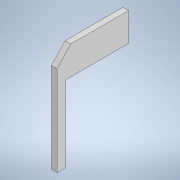
# Autodesk Inventor part: GripperServoAtt
Saved by Autodesk Inventor 2020 (Build 240168000, 168)
## iProperties
Created: 2020-01-21
Part Number: GripperServoAtt
Material: Generic
Document SubType Name: Modeling
Designer: tdmp4
Density: 1 g/cm^3
Appearance: Default
Author: tdmp4
Autodesk Inventor part; units mm, degrees
ref_plane "YZ Plane" through (0, 0, 0) normal (1, 0, 0) x (0, 1, 0)
ref_plane "XZ Plane" through (0, 0, 0) normal (0, 1, 0) x (-1, 0, 0)
ref_plane "XY Plane" through (0, 0, 0) normal (0, 0, 1) x (1, 0, 0)
sketch "Sketch1" plane through (0, 0, 0) normal (1, 0, 0) x (0, 1, 0)
  line L0 (0, 0) -> (25.4, 0)
  line L1 (25.4, 0) -> (25.4, -9.525)
  line L2 (25.4, -9.525) -> (0, -9.525)
  line L3 (0, -9.525) -> (0, 0)
  line L4 (25.4, -9.525) -> (35.5298, -9.525)
  line L5 (35.5298, -9.525) -> (35.5298, -29.845)
  line L6 (25.4, -9.525) -> (25.4, -24.4288)
  line L7 (25.4, -24.4288) -> (25.4, -29.845)
  line L8 (35.5298, -29.845) -> (26.0048, -29.845)
  line L9 (26.0048, -29.845) -> (26.0048, -80.645)
  line L10 (26.0048, -80.645) -> (35.5298, -80.645)
  line L11 (35.5298, -80.645) -> (35.5298, -29.845)
  line L12 (35.5298, -80.645) -> (41.8798, -80.645)
  line L13 (41.8798, -80.645) -> (41.8798, -15.4958)
  line L14 (41.8798, -15.4958) -> (35.5298, -15.4958)
  line L15 (35.5298, -15.4958) -> (35.5298, -80.645)
  line L16 (25.4, 0) -> (35.5298, -9.525)
  line L17 (41.8798, -15.4958) -> (35.5298, -9.525)
  line L18 (26.0048, -29.845) -> (25.4, -29.845)
  line L19 (0, 0) -> (-76.2, 0)
  line L20 (-76.2, 0) -> (-76.2, -9.525)
  line L21 (-76.2, -9.525) -> (0, -9.525)
  line L22 (0, -9.525) -> (0, 0)
  dimension "d0" = 25.4
  dimension "d1" = 9.525
  dimension "d3" = 20.32
  dimension "d11" = 50.8
  dimension "d12" = 6.35
  dimension "d13" = 76.2
  dimension "d14" = 9.525
  constraints: 46 end point, 8 parallel, 6 horizontal, 5 perpendicular, 2 vertical, 1 collinear
  measures "d0" distance of L1.end L2.end
  measures "d1" distance of L2.end L0.start
  measures "d3" distance of L4.end L5.end
  measures "d11" distance of L8.end L9.end
  measures "d12" distance of L14.end L13.end
  measures "d13" distance of L21.end L20.end
  measures "d14" distance of L19.end L20.end
extrude "Extrusion1" add sketch "Sketch1" along normal blind 6.35
sketch "Sketch4" plane through (0, 26.0048, -80.645) normal (0, -1, 0) x (1, 0, 0)
  line L0 (0, 0) -> (0, 65.1492) projected
  line L1 (6.35, 71.12) -> (6.35, 50.8) projected
  line L2 (0, 0) -> (6.35, 0)
  line L3 (6.35, 0) -> (6.35, 71.12)
  line L4 (6.35, 71.12) -> (0, 71.12)
  line L5 (0, 71.12) -> (0, 0)
  point P0 (0, 80.645)
  point P1 (0, 65.1492)
  point P2 (6.35, 50.8)
  constraints: 8 end point, 2 parallel, 1 horizontal, 1 perpendicular
extrude "Extrusion3" add sketch "Sketch4" along normal blind 16.256
body "Solid1"
